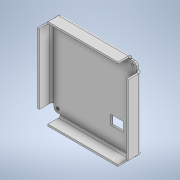
# Autodesk Inventor part: WaageBlechUnterseite
Saved by Autodesk Inventor 2022 (Build 260153000, 153)
## iProperties
Created: 2021-12-03
Part Number: WaageBlechUnterseite
Material: Generic
Document SubType Name: Sheet Metal
Designer: domin
Density: 1 g/cm^3
Sheet Metal Rule: Default_mm
Appearance: Default
Author: domin
Autodesk Inventor part; units mm, degrees
ref_plane "YZ Plane" through (0, 0, 0) normal (1, 0, 0) x (0, 1, 0)
ref_plane "XZ Plane" through (0, 0, 0) normal (0, 1, 0) x (-1, 0, 0)
ref_plane "XY Plane" through (0, 0, 0) normal (0, 0, 1) x (1, 0, 0)
sketch "Sketch1" plane through (0, 0, 0) normal (0, 0, 1) x (1, 0, 0)
  line L0 (55.5, 72) -> (-55.5, 72)
  line L1 (-55.5, 72) -> (-55.5, 65.5)
  line L2 (-55.5, 65.5) -> (-65.5, 65.5)
  line L3 (-65.5, 65.5) -> (-65.5, 55.5)
  line L4 (-65.5, 55.5) -> (-72, 55.5)
  line L5 (-72, 55.5) -> (-72, -55.5)
  line L6 (-72, -55.5) -> (-65.5, -55.5)
  line L7 (-65.5, -55.5) -> (-65.5, -65.5)
  line L8 (-65.5, -65.5) -> (-55.5, -65.5)
  line L9 (-55.5, -65.5) -> (-55.5, -72)
  line L10 (-55.5, -72) -> (55.5, -72)
  line L11 (55.5, -72) -> (55.5, -65.5)
  line L12 (55.5, -65.5) -> (65.5, -65.5)
  line L13 (65.5, -65.5) -> (65.5, -55.5)
  line L14 (65.5, -55.5) -> (72, -55.5)
  line L15 (72, -55.5) -> (72, 55.5)
  line L16 (72, 55.5) -> (65.5, 55.5)
  line L17 (65.5, 55.5) -> (65.5, 65.5)
  line L18 (65.5, 65.5) -> (55.5, 65.5)
  line L19 (55.5, 65.5) -> (55.5, 72)
  point P0 (0, 0)
  dimension "d5" = 144
  dimension "d14" = 144
  dimension "d15" = 72
  dimension "d16" = 72
  dimension "d28" = 10
  dimension "d30" = 10
  dimension "d31" = 10
  dimension "d32" = 111
  dimension "d33" = 111
  measures "d5" distance between parallel lines of L15 L5
  measures "d14" distance between parallel lines of L10 L0
  measures "d15" distance from line of point (0, 0) L5
  measures "d16" distance from line of point (0, 0) L0
  measures "d28" distance of L11.end L12.end
  measures "d30" distance of L6.end L7.end
  measures "d31" distance of L7.end L8.end
  measures "d32" distance between parallel lines of L9 L11
  measures "d33" distance between parallel lines of L4 L6
extrude "Plate1" add sketch "Sketch1" along normal blind 3
sketch "Sketch2" plane through (-69, -55.5, 0) normal (-1, 0, 0) x (0, -1, 0)
  line L0 (-111, 0) -> (0, 0)
  line L1 (0, 0) -> (0, 22.5)
  line L2 (0, 22.5) -> (-111, 22.5)
  line L3 (-111, 22.5) -> (-111, 0)
  constraints: 6 end point, 1 horizontal, 1 perpendicular, 1 vertical
edge flange "Flange1" height 22.5 angle 90 thickness 3 bend radius 3 thickness toward (-1, 0, 0) relief tear relief width 3 relief depth 0 corner gap 3 corner form 0 edges at (-72, 0, 3) (0, -72, 3) (72, 0, 3) (0, 72, 3) wall of the first edge with corners at (-69, 55.5, 0) (-69, -55.5, 0) (-69, -55.5, 22.5) (-69, 55.5, 22.5)
bend "Bend1"
corner "Corner1"
sketch "Sketch3" plane through (0, 0, 3) normal (0, 0, 1) x (1, 0, 0)
  line L0 (59.5, -59.5) -> (-59.5, -59.5)
  line L1 (-59.5, -59.5) -> (-59.5, 59.5)
  line L2 (-59.5, 59.5) -> (59.5, 59.5)
  line L3 (59.5, 59.5) -> (59.5, -59.5)
  circle A0 centre (59.5, -59.5) radius 3
  point P0 (0, 0)
  dimension "d34" = 119
  dimension "d35" = 119
  dimension "d36" = 59.5
  dimension "d37" = 59.5
  dimension "d38" = 6
  constraints: 8 end point, 2 parallel, 1 centre point, 1 coincident, 1 horizontal, 1 perpendicular
  measures "d34" distance of L2.end L0.start
  measures "d35" distance of L0.start L0.end
  measures "d36" distance from line of L3 point (0, 0)
  measures "d37" distance from line of point (0, 0) L0
  measures "d38" diameter of A0
hole "Hole1" at (59.5, -59.5, 3) at (-59.5, -59.5, 3) at (-59.5, 59.5, 3) at (59.5, 59.5, 3) direction (0, 0, -1) diameter 4.917 end through all thread size "M6x1" class "6H" standard "ISO Metric profile"
fillet "Corner Round1" radius 5 4 edges at (65.5, -65.5, 1.5) (65.5, 65.5, 1.5) (-65.5, 65.5, 1.5) (-65.5, -65.5, 1.5)
sketch "Sketch4" plane through (0, 0, 3) normal (0, 0, 1) x (1, 0, 0)
  line L0 (45, -25) -> (25, -25)
  line L1 (25, -25) -> (25, -40)
  line L2 (25, -40) -> (45, -40)
  line L3 (45, -40) -> (45, -25)
  point P0 (0, 0)
  dimension "d47" = 20
  dimension "d48" = 15
  dimension "d49" = 25
  dimension "d50" = 25
  constraints: 8 end point, 2 parallel, 1 horizontal, 1 perpendicular
  measures "d47" distance of L0.start L0.end
  measures "d48" distance of L2.end L0.start
  measures "d49" distance from line of point (0, 0) L1
  measures "d50" distance from line of point (0, 0) L0
extrude "Cut1" cut sketch "Sketch4" against normal blind 3
equation "\"d36\" = 0.5 * d34"
equation "\"d37\" = 0.5 * d35"
equation "\"d40\" = Thickness"
equation "\"d44\" = Thickness"
equation "\"d51\" = Thickness"
equation "\"d17\" = Thickness"
equation "\"d18\" = BendReliefWidth"
equation "\"d20\" = MinimumRemnant"
equation "\"d21\" = TransitionRadius"
equation "\"d24\" = BendRadius"
equation "\"d25\" = CornerReliefSize"
equation "\"d26\" = GapSize"
equation "\"d27\" = JacobiRadiusSize"
equation "\"d15\" = 0.5 * d5"
equation "\"d16\" = 0.5 * d14"
equation "\"BendRadius\" = Thickness"
equation "\"BendReliefWidth\" = Thickness"
equation "\"BendReliefDepth\" = 0.5 * Thickness"
equation "\"CornerReliefSize\" = 4 * Thickness"
equation "\"MinimumRemnant\" = 2 * Thickness"
equation "\"TransitionRadius\" = BendRadius"
equation "\"JacobiRadiusSize\" = BendRadius"
equation "\"GapSize\" = Thickness"
equation "\"Thickness\" = 3"
body "Solid1"
